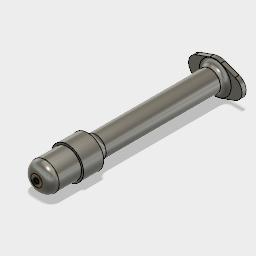
FluxPlunger (Autodesk Fusion 360 design; units mm, degrees)
Autodesk Fusion 360 part; units mm, degrees
note: some values were not read from the file. Set by a fixed rule: which sketch regions a step uses.
sketch "Sketch1" plane through (0, 0, 0) normal (0, 0, 1) x (1, 0, 0)
  circle A0 centre (0, 0) radius 7.6
  circle A1 centre (0, 0) radius 5
  circle A2 centre (0, 0) radius 3.5
  dimension "d1" = 15.2
  dimension "d10" = 10
  dimension "d11" = 1.5
  measures "d1" diameter of A0
  measures "d10" diameter of A1
extrude "Extrude1" add sketch "Sketch1" along normal blind 9.5 contours A0 | A1 | A2
sketch "Sketch2" plane through (0, 0, 9.5) normal (0, 0, 1) x (1, 0, 0)
  circle A0 centre (0, 0) radius 7.6
  circle A1 centre (0, 0) radius 6.65
  dimension "d4" = 13.3
  measures "d4" diameter of A1
extrude "Extrude2" add sketch "Sketch2" along normal blind 8.5 contours A1
sketch "Sketch3" plane through (0, 0, 18) normal (0, 0, 1) x (1, 0, 0)
  circle A0 centre (0, 0) radius 6.65
extrude "Extrude3" add sketch "Sketch3" along normal blind 6
fillet "Fillet1" radius 4 1 edges at (-6.2, -2.4047, 24)
extrude "Extrude4" add sketch "Sketch1" against normal blind 60 contours A1
fillet "Fillet2" radius 4 1 edges at (-4.6616, -1.8081, 0)
sketch "Sketch4" plane through (0, 0, -60) normal (0, 0, -1) x (-1, 0, 0)
  circle A0 centre (0, 0) radius 3.5
  circle A1 centre (0, 0) radius 5
  circle A2 centre (0, 0) radius 7.6
  circle A3 centre (-7.6, 0.0004) radius 5
  circle A4 centre (7.6, 0) radius 5
  line L0 (-9.3103, 4.6988) -> (-2.5996, 7.1416)
  line L1 (2.6, 7.1414) -> (9.3105, 4.6983)
  line L2 (-9.3108, -4.6978) -> (-2.6004, -7.1413)
  line L3 (9.3105, -4.6983) -> (2.6, -7.1414)
  arc A5 (5.9553, 4.7217) -> (5.9552, -4.7218) centre (0, 0) ccw
  dimension "d15" = 10
  dimension "d16" = 10
  measures "d15" diameter of A3
  measures "d16" diameter of A4
extrude "Extrude5" add sketch "Sketch4" along normal blind 2
fillet "Fillet3" radius 2.5 1 edges at (-4.6616, 1.8081, -60)
sketch "Sketch5" plane through (0, 0, 24) normal (0, 0, 1) x (1, 0, 0)
  circle A0 centre (0, 0) radius 2.65
  circle A1 centre (0, 0) radius 1
  dimension "d20" = 2
  measures "d20" diameter of A1
extrude "Extrude6" cut sketch "Sketch5" against normal blind 129 contours A1
